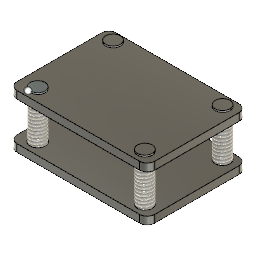
_Chassi Robo Sequidor De Linha.a14916dc-b5e3-4af1-8d63-7f274c80cb8d (Autodesk Fusion 360 design; units mm, degrees)
Autodesk Fusion 360 part; units mm, degrees
sketch "Sketch1" plane through (0, 0, 0) normal (0, 0, 1) x (1, 0, 0)
  line L0 (0, 0) -> (18, 0)
  line L1 (18, 0) -> (18, 13)
  line L2 (18, 13) -> (0, 13)
  line L3 (0, 13) -> (0, 0)
  dimension "d1" = 13
  dimension "d2" = 18
  constraint horizontal L0
  constraint vertical L1
  constraint horizontal L2
  constraint vertical L3
  constraint coincident L0.start L3.end
  measures "d1" distance of L0.start L2.end
  measures "d2" distance of L1.end L2.end
extrude "Extrude1" add sketch "Sketch1" along normal blind 1 makes body 1
hole "Hole1" at (2.1449, 1.5875, 1) direction (0, 0, -1) diameter 2 depth 6 tip angle 118 bodies 1
hole "Hole2" at (16.1882, 1.513, 1) direction (0, 0, -1) diameter 2 depth 6 tip angle 118 bodies 1
hole "Hole3" at (16.2178, 11.6181, 1) direction (0, 0, -1) diameter 2 depth 6 tip angle 118 bodies 1
hole "Hole4" at (1.7862, 11.7662, 1) direction (0, 0, -1) diameter 2 depth 6 tip angle 118 bodies 1
fillet "Fillet1" radius 1 1 edges at (0, 0, 0.5) on bodies 1
fillet "Fillet2" radius 1 1 edges at (18, 0, 0.5) on bodies 1
fillet "Fillet3" radius 1 1 edges at (18, 13, 0.5) on bodies 1
fillet "Fillet4" radius 1 1 edges at (0, 13, 0.5) on bodies 1
copy_body "CopyPasteBodies1" bodies 1 makes body 2
move_body "Move1" bodies 2 to x (1, 0, 0) y (0, 1, 0) z (0, 0, 1) at (0, 0, 6)
sketch "Sketch2" plane through (0, 0, 0) normal (0, 0, 1) x (1, 0, 0)
  circle A0 centre (2.1396, 1.5819) radius 1
  dimension "d21" = 2
  measures "d21" diameter of A0
extrude "Extrude2" cut sketch "Sketch2" along normal blind 6 bodies 1
sketch "Sketch3" plane through (0, 0, 7) normal (0, 0, 1) x (-1, 0, 0)
  arc A0 (-1, -13) -> (0, -12) centre (-1, -12) ccw
  line L0 (0, -12) -> (0, -1)
  arc A1 (0, -1) -> (-1, 0) centre (-1, -1) ccw
  line L1 (-1, 0) -> (-17, 0)
  arc A2 (-17, 0) -> (-18, -1) centre (-17, -1) ccw
  line L2 (-18, -1) -> (-18, -12)
  arc A3 (-18, -12) -> (-17, -13) centre (-17, -12) ccw
  line L3 (-17, -13) -> (-1, -13)
  circle A4 centre (-1.7862, -11.7662) radius 1
  circle A5 centre (-16.2178, -11.6181) radius 1
  circle A6 centre (-16.1882, -1.513) radius 1
  circle A7 centre (-2.1449, -1.5875) radius 1
  circle A8 centre (-2.1449, -1.5875) radius 1
  constraint tangent A7 A8
extrude "Extrude3" add sketch "Sketch3" along normal blind 0.2 separate body contours A7 A8 makes body 3
extrude "Extrude4" add 1 faces at (1.9454, 1.3392, 7) along direction (0, 0, -1) blind 7.2 on bodies 3 bodies 3 1 2
thread "Thread1" "ISO Metric profile 2.0 M2x0.4 6g" major diameter 1.9335 minor diameter 1.478 pitch 0.4 angle 60 resizes the face on face at (1.3493, 2.1933, 2.2667) on bodies 3
thread "Thread2" "ISO Metric profile 2.0 M2x0.4 6g" major diameter 1.9335 minor diameter 1.478 pitch 0.4 angle 60 resizes the face on face at (1.1499, 1.6871, 7.1333) on bodies 3
sketch "Sketch4" plane through (0, 0, 7) normal (0, 0, 1) x (-1, 0, 0)
  arc A0 (-1, -13) -> (0, -12) centre (-1, -12) ccw
  line L0 (0, -12) -> (0, -1)
  arc A1 (0, -1) -> (-1, 0) centre (-1, -1) ccw
  line L1 (-1, 0) -> (-17, 0)
  arc A2 (-17, 0) -> (-18, -1) centre (-17, -1) ccw
  line L2 (-18, -1) -> (-18, -12)
  arc A3 (-18, -12) -> (-17, -13) centre (-17, -12) ccw
  line L3 (-17, -13) -> (-1, -13)
  circle A4 centre (-1.7862, -11.7662) radius 1
  circle A5 centre (-16.2178, -11.6181) radius 1
  circle A6 centre (-16.1882, -1.513) radius 1
  circle A7 centre (-2.1449, -1.5875) radius 0.9668
  circle A8 centre (-16.1882, -1.513) radius 1
  constraint tangent A6 A8
extrude "Extrude5" add sketch "Sketch4" along normal blind 0.2 separate body contours A6 A8 makes body 4
extrude "Extrude6" add 1 faces at (16.1655, 1.1953, 7) along direction (0, 0, -1) blind 7.2 on bodies 4 bodies 4 3
thread "Thread3" "ISO Metric profile 2.0 M2x0.4 6g" major diameter 1.9335 minor diameter 1.478 pitch 0.4 angle 60 resizes the face on face at (1.1829, 1.6838, 3.9333) on face at (15.1932, 1.6125, 4.3333) on bodies 4
thread "Thread4" "ISO Metric profile 2.0 M2x0.4 6g" major diameter 1.9335 minor diameter 1.478 pitch 0.4 angle 60 resizes the face on face at (15.1932, 1.4134, 7.1333) on bodies 4
sketch "Sketch5" plane through (0, 0, 7) normal (0, 0, 1) x (-1, 0, 0)
  arc A0 (-1, -13) -> (0, -12) centre (-1, -12) ccw
  line L0 (0, -12) -> (0, -1)
  arc A1 (0, -1) -> (-1, 0) centre (-1, -1) ccw
  line L1 (-1, 0) -> (-17, 0)
  arc A2 (-17, 0) -> (-18, -1) centre (-17, -1) ccw
  line L2 (-18, -1) -> (-18, -12)
  arc A3 (-18, -12) -> (-17, -13) centre (-17, -12) ccw
  line L3 (-17, -13) -> (-1, -13)
  circle A4 centre (-1.7862, -11.7662) radius 1
  circle A5 centre (-16.2178, -11.6181) radius 1
  circle A6 centre (-16.1882, -1.513) radius 0.9668
  circle A7 centre (-2.1449, -1.5875) radius 0.9668
  circle A8 centre (-16.2178, -11.6181) radius 1
  constraint tangent A5 A8
extrude "Extrude7" add sketch "Sketch5" along normal blind 0.2 separate body contours A5 A8 makes body 5
extrude "Extrude8" add 1 faces at (15.5221, 11.7513, 7) along direction (0, 0, -1) blind 7.2 on bodies 5 bodies 5 4
sketch "Sketch6" plane through (0, 0, 7) normal (0, 0, 1) x (-1, 0, 0)
  arc A0 (-1, -13) -> (0, -12) centre (-1, -12) ccw
  line L0 (0, -12) -> (0, -1)
  arc A1 (0, -1) -> (-1, 0) centre (-1, -1) ccw
  line L1 (-1, 0) -> (-17, 0)
  arc A2 (-17, 0) -> (-18, -1) centre (-17, -1) ccw
  line L2 (-18, -1) -> (-18, -12)
  arc A3 (-18, -12) -> (-17, -13) centre (-17, -12) ccw
  line L3 (-17, -13) -> (-1, -13)
  circle A4 centre (-1.7862, -11.7662) radius 1
  circle A5 centre (-16.2178, -11.6181) radius 1
  circle A6 centre (-16.1882, -1.513) radius 0.9668
  circle A7 centre (-2.1449, -1.5875) radius 0.9668
  circle A8 centre (-1.7862, -11.7662) radius 1
  constraint tangent A4 A8
extrude "Extrude9" add sketch "Sketch6" along normal blind 0.2 separate body contours A4 A8 makes body 6
extrude "Extrude10" add 1 faces at (1.6387, 11.5174, 7) along direction (0, 0, -1) blind 7.2 on bodies 6 bodies 6 5
thread "Thread5" "ISO Metric profile 2.0 M2x0.4 6g" major diameter 1.9335 minor diameter 1.478 pitch 0.4 angle 60 resizes the face on face at (15.2262, 1.6092, 2.6667) on face at (1.1793, 1.6357, 1.8667) on face at (16.4887, 10.6555, 4.3333) on face at (0.7912, 11.8658, 4.3333) on face at (0.7912, 11.8658, 7.1333) on face at (15.2228, 11.7176, 7.1333) on face at (15.2226, 1.4648, 7.0667) on face at (1.1829, 1.6838, 7.0667) on bodies 6
sketch "Sketch7" plane through (0, 0, 7.2) normal (0, 0, 1) x (-1, 0, 0)
  circle A0 centre (-2.1449, -1.5875) radius 0.9668
  line L0 (-2, -0.5) -> (-1.9, -0.5)
  constraint horizontal L0
